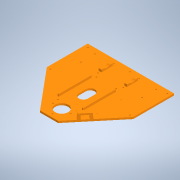
# Autodesk Inventor part: bp_v3
Saved by Autodesk Inventor 2020.3 (Build 243373000, 373)
## iProperties
Created: 2020-06-30
Part Number: bp_v3
Material: PET Plastic
Document SubType Name: Modeling
Designer: Devin
Density: 1.541 g/cm^3
Appearance: Orange
Mass: 167.069 g
Surface Area: 574.42 cm^2
Volume: 108.416 cm^3
Author: Devin
Autodesk Inventor part; units mm, degrees
ref_plane "YZ Plane" through (0, 0, 0) normal (1, 0, 0) x (0, 1, 0)
ref_plane "XZ Plane" through (0, 0, 0) normal (0, 1, 0) x (-1, 0, 0)
ref_plane "XY Plane" through (0, 0, 0) normal (0, 0, 1) x (1, 0, 0)
sketch "Sketch1" plane through (0, 0, 0) normal (0, 1, 0) x (-1, 0, 0)
  line L0 (0, 0) -> (-190, 0)
  line L1 (0, 15) -> (0, 0)
  line L2 (-95, 0) -> (-95, 180)
  line L3 (0, 0) -> (0, 90)
  line L4 (-190, 0) -> (-190, 90)
  line L5 (-95, 180) -> (-75, 180)
  line L6 (-75, 180) -> (0, 90)
  line L7 (-95, 180) -> (-115, 180)
  line L8 (-115, 180) -> (-190, 90)
  dimension "d1" = 190
  dimension "d37" = 180
  dimension "d39" = 20
  dimension "d40" = 20
  constraints: 18 end point, 3 horizontal, 3 vertical, 1 midpoint, 1 point on line
  measures "d1" distance of L0.end L0.start
  measures "d37" distance of L2.start L2.end
  measures "d39" distance of L2.end L5.end
  measures "d40" distance of L2.end L7.end
extrude "Extrusion1" add sketch "Sketch1" along normal blind 4
sketch "Sketch5" plane through (0, 4, 0) normal (0, 1, 0) x (1, 0, 0)
  circle A0 centre (27.5, -12) radius 1.55 projected
  circle A1 centre (27.5, -43) radius 1.55 projected
  circle A2 centre (162.5, -43) radius 1.55 projected
  circle A3 centre (162.5, -12) radius 1.55 projected
  point P0 (0, 0)
extrude "Extrusion2" cut sketch "Sketch5" against normal blind 10
sketch "Sketch6" plane through (0, 4, 0) normal (0, 1, 0) x (1, 0, 0)
  line L0 (64, -39.65) -> (64, -15.35)
  line L1 (190, 0) -> (0, 0) projected
  circle A0 centre (27.5, -43) radius 1.55 projected
  circle A1 centre (27.5, -12) radius 1.55 projected
  line L2 (64, -27.5) -> (64, -15.35)
  line L3 (64, -15.35) -> (70, -15.35)
  line L4 (70, -15.35) -> (70, -39.65)
  line L5 (70, -39.65) -> (64, -39.65)
  line L6 (190, 0) -> (0, 0) projected
  line L7 (126, -39.65) -> (126, -15.35)
  line L8 (126, -15.35) -> (120, -15.35)
  line L9 (120, -15.35) -> (120, -39.65)
  line L10 (120, -39.65) -> (126, -39.65)
  dimension "d131" = 6
  dimension "d132" = 6
  constraints: 18 end point, 1 midpoint
  measures "d131" distance of L0.end L3.end
  measures "d132" distance of L0.start L4.end
extrude "Extrusion3" add sketch "Sketch6" along normal blind 5 contours L0 L3 L4 L5 | L10 L9 L8 L7
sketch "Sketch14" plane through (0, 4, 0) normal (0, 1, 0) x (1, 0, 0)
  line L0 (190, 0) -> (0, 0) projected
  line L1 (0, 0) -> (0, -7.5)
  line L2 (0, 0) -> (0, -15) projected
  line L3 (0, -90) -> (75, -180) projected
  circle A0 centre (7.5, -7.5) radius 1.55
  circle A1 centre (7.5, -90) radius 1.55
  line L4 (75, -180) -> (115, -180) projected
  circle A2 centre (182.5, -7.5) radius 1.55
  circle A3 centre (182.5, -90) radius 1.55
  circle A4 centre (95, -172.5) radius 1.55
  dimension "d68" = 7.5
  dimension "d71" = 3.1
  dimension "d72" = 3.1
  dimension "d74" = 3.1
  constraints: 5 centre point, 2 end point, 1 midpoint
  measures "d68" distance of L0.end L1.end
  measures "d71" diameter of A0
  measures "d72" diameter of A1
  measures "d74" diameter of A4
extrude "Extrusion10" cut sketch "Sketch14" against normal blind 10
sketch "Sketch17" plane through (0, 4, 0) normal (0, 1, 0) x (1, 0, 0)
  circle A0 centre (95, -152.3364) radius 14.25
  line L0 (75, -180) -> (115, -180) projected
  point P0 (0, 0)
  dimension "d101" = 28.5
  dimension "d112" = 27.6636
  constraints: 1 centre point
  measures "d101" diameter of A0
  measures "d112" distance from line of L0 A0.centre
extrude "Extrusion13" cut sketch "Sketch17" against normal through all
sketch "Sketch19" plane through (0, 4, 0) normal (0, 1, 0) x (1, 0, 0)
  circle A0 centre (95, -152.3364) radius 14.25 projected
  circle A1 centre (114.5, -152.3364) radius 1.55
  circle A2 centre (75.5, -152.3364) radius 1.55
  point P0 (0, 0)
  dimension "d108" = 3.1
  dimension "d109" = 3.1
  constraints: 2 centre point
  measures "d108" diameter of A1
  measures "d109" diameter of A2
extrude "Extrusion14" cut sketch "Sketch19" against normal blind 5 contours A1 | A2
sketch "Sketch27" plane through (126, 4, 39.65) normal (1, 0, 0) x (0, 0, -1)
  circle A0 centre (12.15, 14.9) radius 2 projected
  circle A1 centre (12.15, 14.9) radius 12.15 projected
  arc A2 (5.1064, 5) -> (19.1936, 5) centre (12.15, 14.9) ccw
  line L0 (0, 5) -> (24.3, 5) projected
  line L1 (5.1064, 5) -> (19.1936, 5)
  point P0 (39.65, -4)
  point P1 (5.1064, 5)
  constraints: 2 end point, 2 point on circle, 2 point on line, 1 centre point, 1 coincident, 1 concentric
extrude "Extrusion18" cut sketch "Sketch27" against normal through all contours L0 A1 picked at (10.6816, 4.5256)
sketch "Sketch28" plane through (0, 4, 0) normal (0, 1, 0) x (1, 0, 0)
  circle A0 centre (67, -44.8593) radius 1.5 projected
  circle A1 centre (123, -44.8593) radius 1.5 projected
  circle A2 centre (123.1217, -10.1201) radius 1.5 projected
  circle A3 centre (67.1217, -10.1201) radius 1.5 projected
  circle A4 centre (67.1217, -10.1201) radius 1.55
  circle A5 centre (123.1217, -10.1201) radius 1.55
  circle A6 centre (123, -44.8593) radius 1.55
  circle A7 centre (67, -44.8593) radius 1.55
  point P0 (0, 0)
  dimension "d135" = 3.1
  dimension "d136" = 3.1
  dimension "d137" = 3.1
  dimension "d138" = 3.1
  constraints: 4 centre point, 4 coincident
  measures "d135" diameter of A4
  measures "d136" diameter of A5
  measures "d137" diameter of A6
  measures "d138" diameter of A7
extrude "Extrusion19" cut sketch "Sketch28" against normal blind 10 contours A0 | A1 | A2 | A3
sketch "Sketch29" plane through (0, 4, 0) normal (0, 1, 0) x (1, 0, 0)
  circle A0 centre (7.5, -7.5) radius 1.55 projected
  circle A1 centre (182.5, -7.5) radius 1.55 projected
  circle A2 centre (100, -7.5) radius 1.55
  line L0 (0, 0) -> (0, -90) projected
  dimension "d141" = 3.1
  dimension "d194" = 100
  constraints: 1 centre point
  measures "d141" diameter of A2
  measures "d194" distance from line of A2.centre L0
extrude "Extrusion20" cut sketch "Sketch29" against normal blind 10 contours A2
sketch "Sketch30" plane through (0, 4, 0) normal (0, 1, 0) x (1, 0, 0)
  circle A0 centre (100, -7.5) radius 1.55 projected
  line L0 (120.6, -60.7864) -> (120.6, -133.0864)
  line L1 (69.4, -60.7864) -> (69.4, -133.0864)
  circle A1 centre (95, -152.3364) radius 14.25 projected
  line L2 (120.6, -133.0864) -> (69.4, -133.0864)
  line L3 (120.6, -60.7864) -> (69.4, -60.7864)
  line L4 (69.4, -60.7864) -> (69.4, -133.0864)
  line L5 (120.6, -60.7864) -> (120.6, -133.0864)
  line L6 (69.4, -129.6517) -> (69.4, -60.7864)
  line L7 (120.6, -60.7864) -> (123, -60.7864)
  line L8 (123, -60.7864) -> (123, -133.0864)
  line L9 (123, -133.0864) -> (120.6, -133.0864)
  line L10 (120.6, -133.0864) -> (120.6, -60.7864)
  line L11 (69.4, -60.7864) -> (69.4, -133.0864)
  line L12 (69.4, -133.0864) -> (67, -133.0864)
  line L13 (67, -133.0864) -> (67, -60.7864)
  line L14 (67, -60.7864) -> (69.4, -60.7864)
  point P0 (0, 0)
  dimension "d148" = 51.2
  dimension "d149" = 72.3
  dimension "d151" = 2.4
  dimension "d152" = 2.4
  constraints: 30 end point, 6 perpendicular, 4 parallel, 1 horizontal
  measures "d148" distance between parallel lines of L0 L1
  measures "d149" distance of L0.start L0.end
  measures "d151" distance of L8.end L9.end
  measures "d152" distance of L1.end L12.end
extrude "Extrusion21" add sketch "Sketch30" along normal blind 5 contours L7 L8 L9 L0 | L1 L12 L13 L14
sketch "Sketch31" plane through (0, 4, 0) normal (0, 1, 0) x (1, 0, 0)
  line L0 (123, -60.7864) -> (123, -133.0864) projected
  line L1 (128, -73.8364) -> (160, -73.8364)
  line L2 (160, -73.8364) -> (160, -120.0364)
  line L3 (160, -120.0364) -> (128, -120.0364)
  line L4 (128, -120.0364) -> (128, -73.8364)
  line L5 (144, -73.8364) -> (144, -70.8364)
  line L6 (144, -120.0364) -> (144, -123.0364)
  circle A0 centre (144, -70.8364) radius 1
  circle A1 centre (144, -123.0364) radius 1
  point P0 (0, 0)
  dimension "d156" = 32
  dimension "d157" = 46.2
  dimension "d158" = 5
  dimension "d159" = 3
  dimension "d160" = 3
  dimension "d161" = 2
  dimension "d162" = 2
  constraints: 12 end point, 2 centre point, 2 coincident, 2 midpoint, 2 parallel, 2 vertical, 1 horizontal, 1 perpendicular
  measures "d156" distance of L1.start L1.end
  measures "d157" distance of L1.end L2.end
  measures "d158" distance between parallel lines of L4 L0
  measures "d159" distance of L5.start L5.end
  measures "d160" distance of L6.start L6.end
  measures "d161" diameter of A0
  measures "d162" diameter of A1
extrude "Extrusion22" cut sketch "Sketch31" against normal blind 2 contours A0 | A1
sketch "Sketch33" plane through (190, 0, 90) normal (0.7682, 0, 0.6402) x (0.6402, 0, -0.7682)
  line L0 (-117.1537, 0) -> (-117.1537, 4) projected
  line L1 (-117.1537, 4) -> (-82.1537, 4)
  line L2 (-117.1537, 4) -> (0, 4) projected
  line L3 (-82.1537, 4) -> (-82.1537, 12.45)
  line L4 (-82.1537, 12.45) -> (-67.6537, 12.45)
  line L5 (-67.6537, 12.45) -> (-67.6537, 4)
  line L6 (-82.1537, 4) -> (-87.1537, 4)
  line L7 (-87.1537, 4) -> (-87.1537, 16)
  line L8 (-87.1537, 16) -> (-62.6537, 16)
  line L9 (-62.6537, 16) -> (-62.6537, 4)
  point P0 (-52.4951, 0)
  dimension "d171" = 35
  dimension "d172" = 8.45
  dimension "d173" = 14.5
  dimension "d174" = 5
  dimension "d175" = 12
  dimension "d176" = 24.5
  constraints: 16 end point, 4 perpendicular, 4 point on line, 1 horizontal, 1 vertical
  measures "d171" distance of L0.end L1.end
  measures "d172" distance of L1.end L3.end
  measures "d173" distance of L3.end L4.end
  measures "d174" distance of L1.end L6.end
  measures "d175" distance of L6.end L7.end
  measures "d176" distance of L7.end L8.end
extrude "Extrusion24" add sketch "Sketch33" against normal blind 9 contours L7 L8 L9 L2 L5 L4 L3 L1
fillet "Fillet1" radius 2 1 edges at (130.7485, 4, 154.0725)
fillet "Fillet2" radius 2 1 edges at (146.4331, 4, 135.2511)
sketch "Sketch34" plane through (0, 4, 0) normal (0, 1, 0) x (1, 0, 0)
  line L0 (85, -79.4364) -> (105, -79.4364)
  line L1 (105, -79.4364) -> (105, -114.4364)
  line L2 (105, -114.4364) -> (85, -114.4364)
  line L3 (69.4, -60.7864) -> (69.4, -133.0864) projected
  line L4 (120.6, -60.7864) -> (120.6, -133.0864) projected
  line L5 (85, -79.4364) -> (85, -114.4364)
  point P0 (0, 0)
  dimension "d181" = 20
  dimension "d182" = 35
  constraints: 8 end point, 1 horizontal, 1 parallel, 1 perpendicular, 1 vertical
  measures "d181" distance of L0.start L0.end
  measures "d182" distance of L0.end L1.end
extrude "Extrusion25" cut sketch "Sketch34" against normal blind 10
fillet "Fillet3" radius 10 1 edges at (85, 2, 79.4364)
fillet "Fillet4" radius 10 3 edges at (105, 2, 114.4364) (105, 2, 79.4364) (85, 2, 114.4364)
sketch "Sketch35" plane through (0, 4, 0) normal (0, 1, 0) x (1, 0, 0)
  circle A0 centre (116.6, -54.3864) radius 1.5 projected
  circle A1 centre (73.4, -54.3864) radius 1.5 projected
  circle A2 centre (73.4, -139.4864) radius 1.5 projected
  circle A3 centre (116.6, -139.4864) radius 1.5 projected
  circle A4 centre (73.4, -54.3864) radius 1.55
  circle A5 centre (116.6, -54.3864) radius 1.55
  circle A6 centre (116.6, -139.4864) radius 1.55
  circle A7 centre (73.4, -139.4864) radius 1.55
  point P0 (0, 0)
  dimension "d188" = 3.1
  dimension "d189" = 3.1
  dimension "d190" = 3.1
  dimension "d191" = 3.1
  constraints: 4 centre point, 4 coincident
  measures "d188" diameter of A4
  measures "d189" diameter of A5
  measures "d190" diameter of A6
  measures "d191" diameter of A7
extrude "Extrusion26" cut sketch "Sketch35" against normal through all contours A0 | A1 | A2 | A3
body "Solid1"
